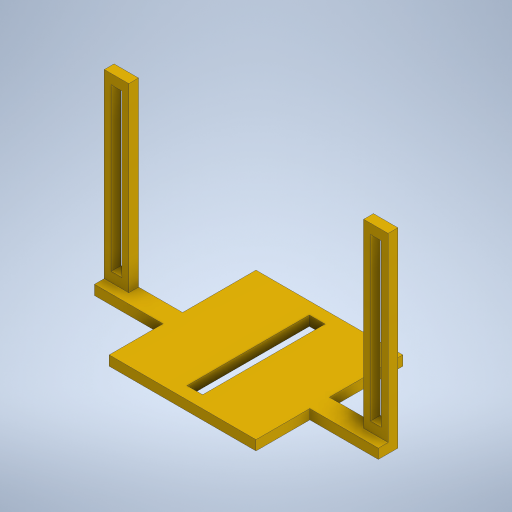
# Autodesk Inventor part: bobbin_support
Saved by Autodesk Inventor 2024 (Build 280153000, 153)
## iProperties
Created: 2022-10-04
Part Number: bobbin_support
Material: Generic
Document SubType Name: Modeling
Designer: gaiadaprato
Density: 1 g/cm^3
Appearance: Default
Author: gaiadaprato
Autodesk Inventor part; units mm, degrees
ref_plane "YZ Plane" through (0, 0, 0) normal (1, 0, 0) x (0, 1, 0)
ref_plane "XZ Plane" through (0, 0, 0) normal (0, 1, 0) x (-1, 0, 0)
ref_plane "XY Plane" through (0, 0, 0) normal (0, 0, 1) x (1, 0, 0)
sketch "Sketch2" plane through (0, 0, 0) normal (0, 1, 0) x (-1, 0, 0)
  line L0 (0, 0) -> (-30, 0)
  line L1 (-30, 0) -> (-30, -30)
  line L2 (-30, -30) -> (0, -30)
  line L3 (0, -30) -> (0, 0)
  line L4 (0, 0) -> (-30, 0)
  line L5 (-30, 0) -> (-30, -2)
  line L6 (0, -2) -> (0, 0)
  line L7 (0, -30) -> (-30, -30)
  line L8 (-30, -30) -> (-30, -44)
  line L9 (0, -44) -> (0, -30)
  point P0 (0, 0)
  dimension "d0" = 30
  dimension "d1" = 30
  constraints: 20 end point, 4 parallel, 3 horizontal, 3 perpendicular, 2 point on line
  measures "d0" distance of L2.end L0.start
  measures "d1" distance of L0.end L0.start
extrude "Extrusion2" add sketch "Sketch2" against normal blind 2
sketch "Sketch5" plane through (0, 0, 0) normal (0, 1, 0) x (1, 0, 0)
  line L0 (13.4, 2.5) -> (16.6, 2.5)
  line L1 (16.6, 2.5) -> (16.6, 27.5)
  line L2 (16.6, 27.5) -> (13.4, 27.5)
  line L3 (13.4, 27.5) -> (13.4, 2.5)
  line L4 (30, 30) -> (0, 30) projected
  line L5 (0, 30) -> (0, 0) projected
  line L6 (30, 0) -> (30, 30) projected
  point P0 (15, 2.5)
  point P1 (15, 27.5)
  dimension "d21" = 25
  dimension "d25" = 3.2
  dimension "d26" = 2.5
  dimension "d56" = 15
  constraints: 8 end point, 2 midpoint, 2 parallel, 1 horizontal, 1 perpendicular
  measures "d21" distance of L2.end L0.start
  measures "d25" distance of L0.start L0.end
  measures "d26" distance from line of L4 point (15, 27.5)
  measures "d56" distance from line of L6 point (15, 27.5)
extrude "Extrusion5" cut sketch "Sketch5" against normal through all
sketch "Sketch6" plane through (0, 0, -30) normal (-1, 0, 0) x (0, 0, 1)
  line L0 (30, 0) -> (0, 0) projected
  line L1 (0, -2) -> (30, -2) projected
  line L2 (15, 0) -> (19, 0)
  line L3 (19, 0) -> (19, -2)
  line L4 (19, -2) -> (15, -2)
  line L5 (15, -2) -> (15, 0)
  line L6 (0, 0) -> (0, -2) projected
  point P0 (0, -1)
  point P1 (15, -1)
  point P2 (15, 0)
  dimension "d28" = 15
  dimension "d29" = 4
  dimension "d30" = 2
  constraints: 8 end point, 4 midpoint, 2 parallel, 1 horizontal, 1 perpendicular, 1 point on line
  measures "d28" distance of point (0, -1) point (15, -1)
  measures "d29" distance of L2.end point (15, 0)
  measures "d30" distance of L3.end L2.end
extrude "Extrusion6" add sketch "Sketch6" along normal blind 14 contours L3 L1 L5 L0
sketch "Sketch7" plane through (30, 0, 0) normal (1, 0, 0) x (0, 0, -1)
  line L0 (0, 0) -> (30, 0) projected
  line L1 (30, -2) -> (0, -2) projected
  line L2 (11, 0) -> (15, 0)
  line L3 (15, 0) -> (15, -2)
  line L4 (15, -2) -> (11, -2)
  line L5 (11, -2) -> (11, 0)
  line L6 (30, 0) -> (30, -2) projected
  point P0 (30, -1)
  point P1 (15, -1)
  point P2 (15, -2)
  dimension "d33" = 15
  dimension "d34" = 4
  constraints: 8 end point, 4 midpoint, 2 parallel, 1 horizontal, 1 perpendicular, 1 point on line
  measures "d33" distance of point (30, -1) point (15, -1)
  measures "d34" distance of L4.end point (15, -2)
extrude "Extrusion7" add sketch "Sketch7" along normal blind 14 contours L0 L3 L1 L5
sketch "Sketch8" plane through (0, 0, 0) normal (0, 1, 0) x (1, 0, 0)
  line L0 (-14, 15) -> (-14, 11) projected
  line L1 (-14, 15) -> (-9, 15)
  line L2 (-9, 15) -> (-9, 13)
  line L3 (-9, 13) -> (-14, 13)
  line L4 (-14, 13) -> (-14, 15)
  line L5 (30, 15) -> (44, 15) projected
  line L6 (44, 15) -> (39, 15)
  line L7 (39, 15) -> (39, 13)
  line L8 (39, 13) -> (44, 13)
  line L9 (44, 13) -> (44, 15)
  point P0 (0, 0)
  point P1 (39, 15)
  point P2 (-14, 13)
  dimension "d37" = 5
  dimension "d38" = 2
  dimension "d39" = 5
  dimension "d40" = 2
  constraints: 16 end point, 4 parallel, 2 horizontal, 2 perpendicular
  measures "d37" distance of L2.end L3.end
  measures "d38" distance of L1.end L2.end
  measures "d39" distance of L8.end L7.end
  measures "d40" distance of L7.end L6.end
extrude "Extrusion8" add sketch "Sketch8" along normal blind 37
sketch "Sketch9" plane through (-14, 0, -13) normal (0, 0, 1) x (1, 0, 0)
  line L0 (3.6, 35) -> (1.4, 35)
  line L1 (1.4, 35) -> (1.4, 2)
  line L2 (1.4, 2) -> (3.6, 2)
  line L3 (3.6, 2) -> (3.6, 35)
  line L4 (0, 37) -> (5, 37) projected
  line L5 (14, 0) -> (0, 0) projected
  line L6 (5, 0) -> (5, 37) projected
  line L7 (0, 0) -> (0, 37) projected
  line L8 (58, 0) -> (58, 37) projected
  line L9 (53, 0) -> (53, 37) projected
  line L10 (54.4, 35) -> (56.6, 35)
  line L11 (56.6, 35) -> (56.6, 2)
  line L12 (56.6, 2) -> (54.4, 2)
  line L13 (54.4, 2) -> (54.4, 35)
  line L14 (53, 37) -> (58, 37) projected
  line L15 (44, 0) -> (58, 0) projected
  point P0 (2.5, 37)
  point P1 (2.5, 35)
  point P2 (2.5, 2)
  point P3 (5, 18.5)
  point P4 (3.6, 18.5)
  point P5 (0, 18.5)
  point P6 (1.4, 18.5)
  point P7 (55.5, 37)
  point P8 (55.5, 35)
  point P9 (55.5, 2)
  dimension "d43" = 2
  dimension "d44" = 2
  dimension "d45" = 1.4
  dimension "d46" = 1.4
  dimension "d47" = 2.2
  dimension "d50" = 1.4
  dimension "d51" = 1.4
  dimension "d52" = 2
  dimension "d53" = 2
  constraints: 16 end point, 10 midpoint, 4 parallel, 2 horizontal, 2 perpendicular
  measures "d43" distance of point (2.5, 37) point (2.5, 35)
  measures "d44" distance from line of L5 point (2.5, 2)
  measures "d45" distance of point (5, 18.5) point (3.6, 18.5)
  measures "d46" distance of point (0, 18.5) point (1.4, 18.5)
  measures "d47" distance between parallel lines of L3 L1
  measures "d50" distance between parallel lines of L9 L13
  measures "d51" distance between parallel lines of L8 L11
  measures "d52" distance of point (55.5, 37) point (55.5, 35)
  measures "d53" distance from line of L15 point (55.5, 2)
extrude "Extrusion9" cut sketch "Sketch9" against normal through all contours L3 L2 L1 L0 | L10 L11 L12 L13
body "Solid2"
